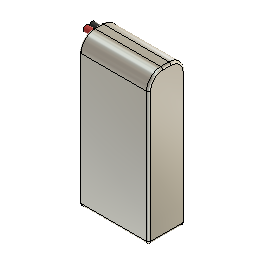
circuit_attachment_fusion (Autodesk Fusion 360 archive; units mm, degrees)
design "Battery v2"
Autodesk Fusion 360 part; units mm, degrees
sketch "Sketch1" plane through (0, 0, 0) normal (0, 0, 1) x (1, 0, 0)
  line L0 (0, 0) -> (34.2, 0)
  line L1 (34.2, 0) -> (34.2, 18)
  line L2 (34.2, 18) -> (0, 18)
  line L3 (0, 18) -> (0, 0)
  dimension "d1" = 34.2
  dimension "d2" = 18
  constraint horizontal L0
  constraint vertical L1
  constraint horizontal L2
  constraint vertical L3
  constraint coincident L0.start L3.end
  measures "d1" distance of L0.start L0.end
  measures "d2" distance of L0.start L2.end
extrude "Extrude1" add sketch "Sketch1" along normal blind 72.4 makes body 1
fillet "Fillet1" radius 7 2 edges at (17.1, 18, 72.4) (17.1, 0, 72.4) on bodies 1
fillet "Fillet2" radius 1 10 edges at (0, 0, 32.7) (0, 2.0503, 70.3497) (0, 9, 72.4) (0, 15.9497, 70.3497) (0, 18, 32.7) (34.2, 0, 32.7) (34.2, 2.0503, 70.3497) (34.2, 9, 72.4) (34.2, 15.9497, 70.3497) (34.2, 18, 32.7) on bodies 1
fillet "Fillet3" radius 1.5 8 edges at (34.2, 9, 0) (33.9071, 17.7071, 0) (17.1, 18, 0) (0.2929, 17.7071, 0) (0, 9, 0) (0.2929, 0.2929, 0) (17.1, 0, 0) (33.9071, 0.2929, 0) on bodies 1
sketch "Sketch2" plane through (0, 0, 0) normal (-1, 0, 0) x (0, -1, 0)
  line L0 (-17, 1.5) -> (-1, 1.5)
  line L1 (-1, 1.5) -> (-1, 65.4)
  arc A0 (-1, 65.4) -> (-7, 71.4) centre (-7, 65.4) ccw
  line L2 (-7, 71.4) -> (-11, 71.4)
  arc A1 (-11, 71.4) -> (-17, 65.4) centre (-11, 65.4) ccw
  line L3 (-17, 65.4) -> (-17, 1.5)
  line L4 (-7, 71.4) -> (-7, 72.4)
  arc A2 (-1, 65.4) -> (-7, 71.4) centre (-7, 65.4) ccw
  line L5 (-1, 65.4) -> (0, 65.4)
  arc A3 (0, 65.4) -> (-7, 72.4) centre (-7, 65.4) ccw
  line L6 (-11, 71.4) -> (-11, 72.4)
  line L7 (-11, 71.4) -> (-7, 71.4)
  line L8 (-7, 71.4) -> (-7, 72.4)
  line L9 (-7, 72.4) -> (-11, 72.4)
  line L10 (-17, 65.4) -> (-18, 65.4)
  arc A4 (-11, 71.4) -> (-17, 65.4) centre (-11, 65.4) ccw
  line L11 (-11, 71.4) -> (-11, 72.4)
  arc A5 (-11, 72.4) -> (-18, 65.4) centre (-11, 65.4) ccw
  circle A6 centre (-7.4912, 69.8818) radius 1.425
  circle A7 centre (-10.5088, 69.8818) radius 1.425
  dimension "d11" = 2.85
  measures "d11" diameter of A6
extrude "Extrude2" add sketch "Sketch2" along normal blind 4 separate body contours A6 makes body 2
extrude "Extrude3" add sketch "Sketch2" along normal blind 4 separate body contours A7 makes body 3
sketch "Sketch3" plane through (0, 0, 0) normal (0, 0, -1) x (1, 0, 0)
  line L0 (32.7, -16.5) -> (32.7, -1.5)
  line L1 (32.7, -1.5) -> (1.5, -1.5)
  line L2 (1.5, -1.5) -> (1.5, -16.5)
  line L3 (1.5, -16.5) -> (32.7, -16.5)
  line L4 (33.2, 0) -> (1, 0)
  line L5 (34.2, -17) -> (34.2, -1)
  line L6 (1, -18) -> (33.2, -18)
  line L7 (0, -1) -> (0, -17)
  line L8 (0, -1) -> (0, 0)
  line L9 (0, 0) -> (1, 0)
  line L10 (33.2, -18) -> (34.2, -18)
  line L11 (34.2, -17) -> (34.2, -18)
  line L12 (0, 0) -> (34.2, 0)
  line L13 (34.2, 0) -> (34.2, -18)
  line L14 (34.2, -18) -> (0, -18)
  line L15 (0, -18) -> (0, 0)
  constraint coincident L7.start L8.start
  constraint parallel L7 L8
  constraint coincident L4.end L9.end
  constraint perpendicular L7 L9
  constraint coincident L6.end L10.start
  constraint parallel L6 L10
  constraint coincident L5.start L11.start
  constraint parallel L5 L11
  constraint horizontal L12
  constraint vertical L13
  constraint horizontal L14
  constraint vertical L15
